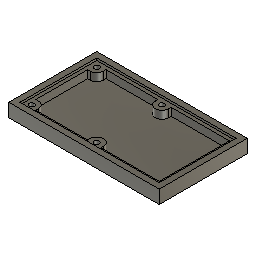
baseplate controller (Autodesk Fusion 360 design; units mm, degrees)
Autodesk Fusion 360 part; units mm, degrees
sketch "Skizze1" plane through (0, 0, 0) normal (0, 0, 1) x (1, 0, 0)
  line L0 (33.75, -19.75) -> (-33.75, -19.75)
  line L1 (-33.75, -19.75) -> (-33.75, 19.75)
  line L2 (-33.75, 19.75) -> (33.75, 19.75)
  line L3 (33.75, 19.75) -> (33.75, -19.75)
  line L4 (33.75, -19.75) -> (-33.75, 19.75) construction
  line L5 (-33.75, -19.75) -> (33.75, 19.75) construction
  dimension "d1" = 67.5
  dimension "d2" = 39.5
  constraint horizontal L0
  constraint perpendicular L0 L1
  constraint parallel L0 L2
  constraint parallel L1 L3
  constraint coincident L4 origin
  constraint coincident L5 origin
  measures "d1" distance of L1.end L2.end
  measures "d2" distance of L0.end L1.end
extrude "Extrusion1" add sketch "Skizze1" along normal blind 6
sketch "Skizze2" plane through (0, 0, 6) normal (0, 0, 1) x (-1, 0, 0)
  line L0 (-33.75, -19.75) -> (33.75, -19.75)
  line L1 (33.75, -19.75) -> (33.75, 19.75)
  line L2 (33.75, 19.75) -> (-33.75, 19.75)
  line L3 (-33.75, 19.75) -> (-33.75, -19.75)
  line L4 (31.25, 17.25) -> (-31.25, 17.25)
  line L5 (-31.25, 17.25) -> (-31.25, -17.25)
  line L6 (-31.25, -17.25) -> (31.25, -17.25)
  line L7 (31.25, -17.25) -> (31.25, 17.25)
  line L8 (31.25, 17.25) -> (-31.25, -17.25) construction
  line L9 (-31.25, 17.25) -> (31.25, -17.25) construction
  dimension "d5" = 34.5
  dimension "d6" = 62.5
  constraint horizontal L4
  constraint perpendicular L4 L5
  constraint parallel L4 L6
  constraint parallel L5 L7
  constraint coincident L8 origin
  constraint coincident L9 origin
  measures "d5" distance of L4.start L6.end
  measures "d6" distance of L5.end L6.end
extrude "Extrusion2" cut sketch "Skizze2" against normal blind 1 contours L4 L5 L6 L7
sketch "Skizze3" plane through (0, 0, 5) normal (0, 0, 1) x (-1, 0, 0)
  line L0 (31.25, -17.25) -> (31.25, 17.25)
  line L1 (31.25, 17.25) -> (-31.25, 17.25)
  line L2 (-31.25, 17.25) -> (-31.25, -17.25)
  line L3 (-31.25, -17.25) -> (31.25, -17.25)
  line L4 (29.75, -15.75) -> (-29.75, -15.75)
  line L5 (-29.75, -15.75) -> (-29.75, 15.75)
  line L6 (-29.75, 15.75) -> (29.75, 15.75)
  line L7 (29.75, 15.75) -> (29.75, -15.75)
  line L8 (29.75, -15.75) -> (-29.75, 15.75) construction
  line L9 (-29.75, -15.75) -> (29.75, 15.75) construction
  line L10 (28.605, -14.605) -> (-0.605, -14.605) construction
  line L11 (-0.605, -14.605) -> (-0.605, 14.605) construction
  line L12 (-0.605, 14.605) -> (28.605, 14.605) construction
  line L13 (28.605, 14.605) -> (28.605, -14.605) construction
  line L14 (31.25, -17.25) -> (28.605, -14.605) construction
  line L15 (31.25, 17.25) -> (28.605, 14.605) construction
  line L16 (28.605, -11.605) -> (29.75, -11.605)
  line L17 (25.605, -14.605) -> (25.605, -15.75)
  line L18 (28.605, 11.605) -> (29.75, 11.605)
  line L19 (25.605, 14.605) -> (25.605, 15.75)
  arc A0 (28.605, -11.605) -> (25.605, -14.605) centre (28.605, -14.605) ccw
  arc A1 (25.605, 14.605) -> (28.605, 11.605) centre (28.605, 14.605) ccw
  line L20 (2.395, 14.605) -> (2.395, 15.75)
  line L21 (-3.605, 14.605) -> (-3.605, 15.75)
  line L22 (2.395, -14.605) -> (2.395, -15.75)
  line L23 (-3.605, -14.605) -> (-3.605, -15.75)
  arc A2 (2.395, -14.605) -> (-3.605, -14.605) centre (-0.605, -14.605) ccw
  arc A3 (-3.605, 14.605) -> (2.395, 14.605) centre (-0.605, 14.605) ccw
  dimension "d9" = 1.5
  dimension "d10" = 1.5
  dimension "d13" = 29.21
  dimension "d14" = 29.21
  dimension "d15" = 6
  constraint horizontal L4
  constraint perpendicular L4 L5
  constraint parallel L4 L6
  constraint parallel L5 L7
  constraint coincident L8 origin
  constraint coincident L9 origin
  constraint horizontal L10
  constraint vertical L11
  constraint horizontal L12
  constraint vertical L13
  constraint coincident L0.start L3.end
  constraint coincident L0.end L1.start
  constraint perpendicular L14 L15
  constraint equal L14 L15
  constraint coincident L10.start L13.end
  constraint coincident L10.end L11.start
  constraint coincident L12.end L13.start
  constraint coincident L11.end L12.start
  constraint equal A0 A1
  constraint equal A0 A2
  constraint equal A0 A3
  constraint coincident L13 L16.start
  constraint coincident L7 L16.end
  constraint tangent L16 A0
  constraint coincident L10 L17.start
  constraint coincident L4 L17.end
  constraint tangent L17 A0
  constraint coincident L13 L18.start
  constraint coincident L7 L18.end
  constraint tangent L18 A1
  constraint coincident L12 L19.start
  constraint coincident L6 L19.end
  constraint tangent L19 A1
  constraint coincident L12 L20.start
  constraint coincident L6 L20.end
  constraint tangent L20 A3
  constraint coincident L6 L21.end
  constraint tangent L21 A3
  constraint perpendicular L6 L21
  constraint coincident L10 L22.start
  constraint coincident L4 L22.end
  constraint tangent L22 A2
  constraint coincident L4 L23.end
  constraint tangent L23 A2
  constraint perpendicular L4 L23
  measures "d9" distance of L0 L7
  measures "d10" distance of L3 L4
  measures "d13" distance of L10.start L12.end
  measures "d14" distance of L10.start L10.end
  measures "d15" diameter of A0
extrude "Extrusion3" cut sketch "Skizze3" against normal up to surface (3.5 mm away) contours L4 L5 L6 L7 L16 L17 L18 L19 A0 A1 L20 L21 L22 L23 A2 A3
sketch "Skizze4" plane through (0, 0, 5) normal (0, 0, 1) x (-1, 0, 0)
  line L0 (2.395, 14.605) -> (2.395, 15.75)
  line L1 (2.395, 15.75) -> (25.605, 15.75)
  line L2 (25.605, 15.75) -> (25.605, 14.605)
  arc A0 (25.605, 14.605) -> (28.605, 11.605) centre (28.605, 14.605) ccw
  line L3 (28.605, 11.605) -> (29.75, 11.605)
  line L4 (29.75, 11.605) -> (29.75, -11.605)
  line L5 (29.75, -11.605) -> (28.605, -11.605)
  arc A1 (28.605, -11.605) -> (25.605, -14.605) centre (28.605, -14.605) ccw
  line L6 (25.605, -14.605) -> (25.605, -15.75)
  line L7 (25.605, -15.75) -> (2.395, -15.75)
  line L8 (2.395, -15.75) -> (2.395, -14.605)
  arc A2 (2.395, -14.605) -> (-3.605, -14.605) centre (-0.605, -14.605) ccw
  line L9 (-3.605, -14.605) -> (-3.605, -15.75)
  line L10 (-3.605, -15.75) -> (-29.75, -15.75)
  line L11 (-29.75, -15.75) -> (-29.75, 15.75)
  line L12 (-29.75, 15.75) -> (-3.605, 15.75)
  line L13 (-3.605, 15.75) -> (-3.605, 14.605)
  arc A3 (-3.605, 14.605) -> (2.395, 14.605) centre (-0.605, 14.605) ccw
  line L14 (31.25, -17.25) -> (31.25, 17.25)
  line L15 (31.25, 17.25) -> (-31.25, 17.25)
  line L16 (-31.25, 17.25) -> (-31.25, -17.25)
  line L17 (-31.25, -17.25) -> (31.25, -17.25)
  circle A4 centre (28.605, -14.605) radius 1.15
  circle A5 centre (-0.605, -14.605) radius 1.15
  circle A6 centre (28.605, 14.605) radius 1.15
  circle A7 centre (-0.605, 14.605) radius 1.15
  dimension "d16" = 2.3
  constraint concentric A1 A4
  constraint concentric A2 A5
  constraint concentric A0 A6
  constraint concentric A3 A7
  constraint equal A4 A5
  constraint equal A4 A6
  constraint equal A4 A7
  measures "d16" diameter of A4
extrude "Extrusion4" cut sketch "Skizze4" against normal through all contours A4 | A5 | A6 | A7
sketch "Skizze5" plane through (0, 0, 0) normal (0, 0, -1) x (1, 0, 0)
  circle A0 centre (0.605, -14.605) radius 1.15
  circle A1 centre (-28.605, 14.605) radius 1.15
  circle A2 centre (-28.605, -14.605) radius 1.15
  circle A3 centre (0.605, 14.605) radius 1.15
  line L0 (-33.75, -19.75) -> (33.75, -19.75)
  line L1 (33.75, -19.75) -> (33.75, 19.75)
  line L2 (33.75, 19.75) -> (-33.75, 19.75)
  line L3 (-33.75, 19.75) -> (-33.75, -19.75)
  line L4 (-27.3926, 12.505) -> (-26.1801, 14.605)
  line L5 (-26.1801, 14.605) -> (-27.3926, 16.705)
  line L6 (-27.3926, 16.705) -> (-29.8174, 16.705)
  line L7 (-29.8174, 16.705) -> (-31.0299, 14.605)
  line L8 (-31.0299, 14.605) -> (-29.8174, 12.505)
  line L9 (-29.8174, 12.505) -> (-27.3926, 12.505)
  circle A4 centre (-28.605, 14.605) radius 1.15
  line L10 (-29.8174, -12.505) -> (-31.0299, -14.605)
  line L11 (-31.0299, -14.605) -> (-29.8174, -16.705)
  line L12 (-29.8174, -16.705) -> (-27.3926, -16.705)
  line L13 (-27.3926, -16.705) -> (-26.1801, -14.605)
  line L14 (-26.1801, -14.605) -> (-27.3926, -12.505)
  line L15 (-27.3926, -12.505) -> (-29.8174, -12.505)
  line L16 (1.8174, 12.505) -> (3.0299, 14.605)
  line L17 (3.0299, 14.605) -> (1.8174, 16.705)
  line L18 (1.8174, 16.705) -> (-0.6074, 16.705)
  line L19 (-0.6074, 16.705) -> (-1.8199, 14.605)
  line L20 (-1.8199, 14.605) -> (-0.6074, 12.505)
  line L21 (-0.6074, 12.505) -> (1.8174, 12.505)
  line L22 (-0.6074, -12.505) -> (-1.8199, -14.605)
  line L23 (-1.8199, -14.605) -> (-0.6074, -16.705)
  line L24 (-0.6074, -16.705) -> (1.8174, -16.705)
  line L25 (1.8174, -16.705) -> (3.0299, -14.605)
  line L26 (3.0299, -14.605) -> (1.8174, -12.505)
  line L27 (1.8174, -12.505) -> (-0.6074, -12.505)
  circle A5 centre (0.605, -14.605) radius 1.15
  point P0 (-28.605, 14.605)
  point P1 (-28.605, -14.605)
  point P2 (0.605, 14.605)
  point P3 (0.605, -14.605)
  dimension "d18" = 4.2
  constraint coincident P0 A1.centre
  constraint coincident P1 A2.centre
  constraint coincident P2 A3.centre
  constraint coincident P3 A0.centre
  constraint horizontal L9
  constraint horizontal L21
  constraint horizontal L27
  constraint horizontal L15
  constraint equal L9 L21
  constraint equal L9 L15
  constraint equal L15 L27
  measures "d18" distance of L6 L9
extrude "Extrusion5" cut sketch "Skizze5" against normal blind 2.5 contours L4 L5 L6 L7 L8 L9 | L10 L11 L12 L13 L14 L15 | L16 L17 L18 L19 L20 L21 | L22 L23 L24 L25 L26 L27
equation "d10 = d9"
named bodies: "Control Universal Boden"
